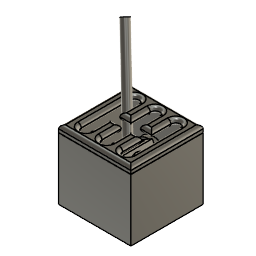
sim shifter v7 (Autodesk Fusion 360 design; units mm, degrees)
Autodesk Fusion 360 part; units mm, degrees
sketch "Sketch1" plane through (0, 0, 0) normal (1, 0, 0) x (0, 1, 0)
  line L0 (10, 18) -> (-10, 18)
  line L1 (-10, 18) -> (-10, 25)
  line L2 (10, 18) -> (10, 25)
  spline S0 degree 2 poles (-10, 25) (0, 18) (10, 25) knots 0 0 0 2.258871 2.258871 2.258871 weights 1 3 1
  line L3 (-22, 25) -> (-10, 25)
  line L4 (22, 25) -> (10, 25)
  line L5 (-16, 25) -> (-16, 20)
  line L6 (16, 25) -> (16, 20)
  spline S1 degree 2 poles (10, 25) (16, 20) (22, 25) knots 0 0 0 1.415097 1.415097 1.415097 weights 1 3 1
  spline S2 degree 2 poles (-22, 25) (-16, 20) (-10, 25) knots 0 0 0 1.415097 1.415097 1.415097 weights 1 3 1
  line L7 (-22, 11) -> (-25, 11)
  line L8 (-25, 11) -> (-25, 25)
  line L9 (-25, 25) -> (-22, 25)
  line L10 (22, 11) -> (22, 25)
  line L11 (-25, 25) -> (-20, 25)
  line L12 (0, 50) -> (0, 54)
  circle A0 centre (0, 50) radius 11
  circle A1 centre (0, 50) radius 4
  circle A2 centre (0, 14.836) radius 4
  line L13 (-22, 11) -> (-22, 25)
  line L14 (22, 11) -> (0, 11)
  line L15 (0, 11) -> (-22, 11)
  line L16 (22, 11) -> (25, 11)
  line L17 (25, 11) -> (25, 25)
  line L18 (25, 25) -> (22, 25)
  line L19 (22, 25) -> (22, 11)
  line L20 (0, 50) -> (7, 50)
  line L21 (7, 50) -> (7, 9.4684)
  line L22 (0, 50) -> (-7, 50)
  line L23 (-7, 50) -> (-7, 9.4684)
  line L24 (-7, 9.4684) -> (7, 9.4684)
  line L25 (-7, 50) -> (7, 50)
  line L26 (7, 50) -> (7, 70)
  line L27 (7, 70) -> (-7, 70)
  line L28 (-7, 70) -> (-7, 50)
  line L29 (-3.9999, 14.8053) -> (4.0001, 14.8053)
  line L30 (4.0001, 14.8053) -> (4.0001, 34.8053)
  line L31 (4.0001, 34.8053) -> (-3.9999, 34.8053)
  line L32 (-3.9999, 34.8053) -> (-3.9999, 14.8053)
  circle A3 centre (0.0001, 34.8053) radius 4
  line L33 (-25, 25) -> (-22, 25)
  line L34 (-22, 25) -> (-22, 65)
  line L35 (-22, 65) -> (-25, 65)
  line L36 (-25, 65) -> (-25, 25)
  line L37 (25, 25) -> (22, 25)
  line L38 (22, 25) -> (22, 65)
  line L39 (22, 65) -> (25, 65)
  line L40 (25, 65) -> (25, 25)
  line L41 (-22, 65) -> (22, 65)
  line L42 (22, 65) -> (22, 35.821)
  line L43 (22, 35.821) -> (-22, 35.821)
  line L44 (-22, 35.821) -> (-22, 65)
  dimension "d7" = 7
  dimension "d8" = 7
  dimension "d12" = 5
  dimension "d13" = 5
  dimension "d76" = 3
  dimension "d77" = 14
  dimension "d120" = 22
  dimension "d121" = 8
  dimension "d122" = 8
  dimension "d123" = 22
  dimension "d124" = 22
  dimension "d127" = 3
  dimension "d128" = 7
  dimension "d131" = 7
  dimension "d132" = 20
  dimension "d133" = 8
  dimension "d134" = 20
  dimension "d143" = 40
  dimension "d144" = 40
  constraint horizontal L0
  constraint perpendicular L0 L1
  constraint perpendicular L0 L2
  constraint perpendicular L1 L3
  constraint perpendicular L2 L4
  constraint midpoint L3 L5.start
  constraint perpendicular L3 L5
  constraint midpoint L4 L6.start
  constraint perpendicular L4 L6
  constraint perpendicular L3 L8
  constraint vertical L10
  constraint horizontal L11
  constraint coincident L12.start A0.centre
  constraint concentric A0 A1
  constraint perpendicular L9 L13
  constraint horizontal L14
  constraint perpendicular L10 L15
  constraint horizontal L16
  constraint vertical L17
  constraint horizontal L18
  constraint vertical L19
  constraint horizontal L20
  constraint vertical L21
  constraint perpendicular L12 L22
  constraint perpendicular L21 L24
  constraint horizontal L25
  constraint vertical L26
  constraint horizontal L27
  constraint vertical L28
  constraint horizontal L29
  constraint vertical L30
  constraint horizontal L31
  constraint vertical L32
  constraint coincident A2 L29.start
  constraint midpoint L31 A3.centre
  constraint coincident L30.end A3
  constraint horizontal L33
  constraint vertical L34
  constraint horizontal L35
  constraint vertical L36
  constraint horizontal L37
  constraint vertical L38
  constraint horizontal L39
  constraint vertical L40
  constraint horizontal L41
  constraint vertical L42
  constraint horizontal L43
  constraint vertical L44
  constraint coincident L38 L42.end
  measures "d7" distance of L0.end L1.end
  measures "d8" distance of L0.start L2.end
  measures "d12" distance of L5.start L5.end
  measures "d13" distance of L6.start L6.end
  measures "d76" distance of L7.start L7.end
  measures "d77" distance of L7.end L8.end
  measures "d120" diameter of A0
  measures "d121" diameter of A1
  measures "d122" diameter of A2
  measures "d123" distance of L10.start L14.end
  measures "d124" distance of L7.start L14.end
  measures "d127" distance of L10.start L16.end
  measures "d128" distance of L12.start L20.end
  measures "d131" distance of L12.start L22.end
  measures "d132" distance of L22.end L27.end
  measures "d133" distance of L29.start L29.end
  measures "d134" distance of L29.end L30.end
  measures "d143" distance of L8.end L35.end
  measures "d144" distance of L17.end L39.end
extrude "Extrude15" add sketch "Sketch1" along normal mid plane 20 contours A0 A1 L20 L21 L22 L23 L25 | A0 A1 L20 L22 L25 L26 L28 | A0 L26 L28 L41 | L26 L27 L28 L41 makes body 1
extrude "Extrude22" add sketch "Sketch1" along normal mid plane 10 contours L0 A2 L14 L21 L30 | L0 S0 L21 L30 | S0 L21 L30 A3 L43 | A2 L14 L15 L21 L23 L24 | L0 A2 L15 L23 L32 | A0 L21 L23 A3 L43 | L0 S0 L23 L32 | S0 L23 L32 A3 L43 bodies 1
extrude "Extrude16" add sketch "Sketch1" along normal mid plane 40 separate body contours L0 L2 S1 L10 L14 L19 L21 | L0 L2 S0 L21 | L0 A2 L14 L21 L30 | L0 S0 L21 L30 | L0 A2 L30 | L0 S0 A2 L30 L32 | L0 A2 L15 L23 L32 | L0 A2 L29 L30 | L0 A2 | L10 L16 L17 L18 L19 L37 | A2 L14 L15 L29 | L18 L37 L38 L39 L40 L42 | L0 A2 L32 | L0 S0 L23 L32 | L0 L1 S0 L23 | L0 L1 S2 L13 L15 L23 | L7 L8 L9 L11 L13 L33 | L9 L11 L33 L34 L35 L36 L44 makes body 2
extrude "Extrude17" cut sketch "Sketch1" along normal mid plane 20.4 contours L0 L2 S1 L10 L14 L19 L21 | L0 L2 S0 L21 | L0 A2 L14 L21 L30 | L0 S0 L21 L30 | L0 A2 L30 | L0 S0 A2 L30 L32 | L0 A2 L15 L23 L32 | L0 A2 L29 L30 | L0 A2 | A2 L14 L15 L29 | L0 A2 L32 | L0 S0 L23 L32 | L0 L1 S0 L23 | L0 L1 S2 L13 L15 L23 bodies 2
extrude "Extrude18" add sketch "Sketch1" along normal blind 10.2 and the other way blind -20 contours A0 L21 L23 A3 L43 | A0 L21 L26 L38 L41 L42 L43 | L18 L37 L38 L39 L40 L42 | A3 L43 | A0 L23 L28 L34 L41 L43 L44 | A0 L26 L28 L41 | L9 L11 L33 L34 L35 L36 L44 bodies 2
extrude "Extrude19" add sketch "Sketch1" along normal blind -10.2 and the other way blind 20 contours A0 L21 L23 A3 L43 | A0 L21 L26 L38 L41 L42 L43 | L18 L37 L38 L39 L40 L42 | A3 L43 | A0 L23 L28 L34 L41 L43 L44 | A0 L26 L28 L41 | L9 L11 L33 L34 L35 L36 L44 bodies 2
sketch "Sketch4" plane through (0, -25, 0) normal (0, -1, 0) x (1, 0, 0)
  circle A0 through (11, 50, -25) (-5.5, 59.5263, -25) (-5.5, 40.4737, -25)
  circle A1 through (20, 50, -25) (-10, 67.3205, -25) (-10, 32.6795, -25)
  circle A2 through (4, 50, -25) (-2, 53.4641, -25) (-2, 46.5359, -25)
  line L0 (0, 50, -25) -> (0, 25, -25)
  line L1 (0, 25, -25) -> (-20, 25, -25)
  line L2 (0, 25, -25) -> (20, 25, -25)
  line L3 (20, 25, -25) -> (45, 25, -25)
  line L4 (-20, 25, -25) -> (-45, 25, -25)
  line L5 (20, 25, -25) -> (30.6066, 35.6066, -25)
  line L6 (20, 25, -25) -> (35, 25, -25) construction
  line L7 (-20, 25, -25) -> (-30.6066, 35.6066, -25)
  line L8 (-20, 25, -25) -> (-35, 25, -25) construction
  spline S0 degree 5 poles (-45, 25, -25) (-44.3564, 25.3564, -25) (-43.0817, 26.0817, -25) (-41.2073, 27.2073, -25) (-38.7846, 28.7846, -25) (-35.8924, 30.8924, -25) (-33.1485, 33.1485, -25) (-30.565, 35.565, -25) (-28.1485, 38.1485, -25) (-25.8924, 40.8924, -25) (-23.7846, 43.7846, -25) (-22.2073, 46.2073, -25) (-21.0817, 48.0817, -25) (-20.3564, 49.3564, -25) (-20, 50, -25) knots 0 0 0 0 0 0 0.1 0.2 0.3 0.4 0.5 0.6 0.7 0.8 0.9 1 1 1 1 1 1
  spline S1 degree 5 poles (20, 50, -25) (20.3564, 49.3564, -25) (21.0817, 48.0817, -25) (22.2073, 46.2073, -25) (23.7846, 43.7846, -25) (25.8924, 40.8924, -25) (28.1485, 38.1485, -25) (30.565, 35.565, -25) (33.1485, 33.1485, -25) (35.8924, 30.8924, -25) (38.7846, 28.7846, -25) (41.2073, 27.2073, -25) (43.0817, 26.0817, -25) (44.3564, 25.3564, -25) (45, 25, -25) knots 0 0 0 0 0 0 0.1 0.2 0.3 0.4 0.5 0.6 0.7 0.8 0.9 1 1 1 1 1 1
  line L9 (45, 25, -25) -> (-45, 25, -25)
  line L10 (-45, 25, -25) -> (-45, 5, -25)
  line L11 (-45, 5, -25) -> (45, 5, -25)
  line L12 (45, 5, -25) -> (45, 25, -25)
  point P0 (0, 50)
  dimension "d153" = 22
  dimension "d154" = 8
  dimension "d155" = 25
  dimension "d156" = 90
  dimension "d157" = 25
  dimension "d159" = 15
  dimension "d160" = 45
  dimension "d161" = 45
  dimension "d162" = 15
  dimension "d171" = 90
  dimension "d172" = 20
extrude "Extrude20" add sketch "Sketch4" along normal blind 25.2 and the other way blind -32 separate body contours A1 | A1 L0 L2 L5 S1 L9 | A1 L0 L1 L7 S0 L9 | L3 L5 S1 L9 | L4 L7 S0 L9 | L1 L2 L3 L4 L9 L10 L11 L12 in plane through (0, 0, 0) normal (0, -1, 0) makes body 3
extrude "Extrude21" add sketch "Sketch4" along normal blind -25.2 and the other way blind 32 separate body contours A1 | A1 L0 L2 L5 S1 L9 | A1 L0 L1 L7 S0 L9 | L3 L5 S1 L9 | L4 L7 S0 L9 | L1 L2 L3 L4 L9 L10 L11 L12 in plane through (0, 0, 0) normal (0, -1, 0) makes body 4
extrude "Extrude23" add sketch "Sketch4" along normal blind 10 from surface at 32 contours L1 L2 L3 L4 L9 L10 L11 L12 in plane through (0, 0, 0) normal (0, -1, 0) bodies 3
extrude "Extrude24" add sketch "Sketch4" against normal blind 10 from surface at -32 contours L1 L2 L3 L4 L9 L10 L11 L12 in plane through (0, 0, 0) normal (0, -1, 0) bodies 4
sketch "Sketch5" plane through (0, 0, 25) normal (0, 0, 1) x (-1, 0, 0)
  line L0 (-45, 32, 10) -> (45, 32, 10)
  line L1 (45, 32, 10) -> (45, 42, 10)
  line L2 (45, 42, 10) -> (-45, 42, 10)
  line L3 (-45, 42, 10) -> (-45, 32, 10)
  line L4 (45, -32, 10) -> (-45, -32, 10)
  line L5 (-45, -32, 10) -> (-45, -42, 10)
  line L6 (-45, -42, 10) -> (45, -42, 10)
  line L7 (45, -42, 10) -> (45, -32, 10)
  line L8 (-45, 25.2, 10) -> (-20, 25.2, 10)
  line L9 (-20, 25.2, 10) -> (-20, 32, 10)
  line L10 (-45, 32, 10) -> (-20, 32, 10)
  line L11 (-45, 32, 10) -> (-45, 25.2, 10)
  line L12 (-20, -25.2, 10) -> (-45, -25.2, 10)
  line L13 (-45, -25.2, 10) -> (-45, -32, 10)
  line L14 (-20, -32, 10) -> (-45, -32, 10)
  line L15 (-20, -32, 10) -> (-20, -25.2, 10)
  line L16 (45, -25.2, 10) -> (20, -25.2, 10)
  line L17 (20, -25.2, 10) -> (20, -32, 10)
  line L18 (45, -32, 10) -> (20, -32, 10)
  line L19 (45, -32, 10) -> (45, -25.2, 10)
  line L20 (20, 25.2, 10) -> (45, 25.2, 10)
  line L21 (45, 25.2, 10) -> (45, 32, 10)
  line L22 (20, 32, 10) -> (45, 32, 10)
  line L23 (20, 32, 10) -> (20, 25.2, 10)
  line L24 (-45, -37, 10) -> (-35, -37, 10)
  line L25 (45, -37, 10) -> (35, -37, 10)
  line L26 (45, 37, 10) -> (35, 37, 10)
  line L27 (-45, 37, 10) -> (-35, 37, 10)
  line L28 (-45, 28.6, 10) -> (-35, 28.6, 10)
  line L29 (45, 28.6, 10) -> (35, 28.6, 10)
  line L30 (45, -28.6, 10) -> (35, -28.6, 10)
  line L31 (-45, -28.6, 10) -> (-35, -28.6, 10)
  dimension "d183" = 10
  dimension "d184" = 10
  dimension "d185" = 10
  dimension "d186" = 10
  dimension "d187" = 10
  dimension "d188" = 10
  dimension "d189" = 10
  dimension "d207" = 10
sketch "Sketch6" plane through (0, 0, 0) normal (0, 0, 1) x (1, 0, 0)
  line L0 (-45, -42) -> (45, -42)
  line L1 (45, -42) -> (45, -32)
  line L2 (45, -32) -> (-45, -32)
  line L3 (45, -32) -> (-45, -32)
  line L4 (-45, -32) -> (-45, -42)
  line L5 (-45, -42) -> (45, -42)
  line L6 (45, 42) -> (-45, 42)
  line L7 (-45, 42) -> (-45, 32)
  line L8 (-45, 32) -> (45, 32)
  line L9 (-45, 32) -> (45, 32)
  line L10 (45, 32) -> (45, 42)
  line L11 (45, 42) -> (-45, 42)
  line L12 (-45, 42) -> (45, 42)
  line L13 (45, 42) -> (45, -42)
  line L14 (45, -42) -> (-45, -42)
  line L15 (-45, -42) -> (-45, 42)
  line L16 (47.5, 47.5) -> (-47.5, 47.5)
  line L17 (-47.5, 47.5) -> (-47.5, -47.5)
  line L18 (-47.5, -47.5) -> (47.5, -47.5)
  line L19 (47.5, -47.5) -> (47.5, 47.5)
  line L20 (47.5, 47.5) -> (-47.5, -47.5) construction
  line L21 (-47.5, 47.5) -> (47.5, -47.5) construction
  line L22 (52.5, -52.5) -> (-52.5, -52.5)
  line L23 (-52.5, -52.5) -> (-52.5, 52.5)
  line L24 (-52.5, 52.5) -> (52.5, 52.5)
  line L25 (52.5, 52.5) -> (52.5, -52.5)
  line L26 (52.5, -52.5) -> (-52.5, 52.5) construction
  line L27 (-52.5, -52.5) -> (52.5, 52.5) construction
  line L28 (-45, -32) -> (-45, -42)
  line L29 (45, -42) -> (45, -32)
  line L30 (45, 32) -> (45, 42)
  line L31 (-45, 42) -> (-45, 32)
  dimension "d197" = 95
  dimension "d198" = 95
  dimension "d199" = 105
  dimension "d200" = 105
  constraint horizontal L12
  constraint vertical L13
  constraint horizontal L14
  constraint vertical L15
  constraint coincident L0.end L1.start
  constraint coincident L6.end L7.start
  constraint horizontal L16
  constraint perpendicular L16 L17
  constraint parallel L16 L18
  constraint parallel L17 L19
  constraint coincident L20 origin
  constraint coincident L21 origin
  constraint horizontal L22
  constraint perpendicular L22 L23
  constraint parallel L22 L24
  constraint parallel L23 L25
  constraint coincident L26 origin
  constraint coincident L27 origin
  measures "d197" distance of L17.end L18.end
  measures "d198" distance of L16.end L17.end
  measures "d199" distance of L23.end L24.end
  measures "d200" distance of L22.end L23.end
extrude "Extrude25" add sketch "Sketch6" along normal blind 5 separate body contours L0 L1 L2 L3 L4 L5 L13 L14 L15 L28 L29 | L2 L3 L8 L9 L13 L15 | L6 L7 L8 L9 L10 L11 L12 L13 L15 L30 L31 | L16 L17 L18 L19 | L22 L23 L24 L25 makes body 5
hole "Hole2" at (35, 37, 35) at (35, 28.6, 35) at (35, -28.6, 35) at (35, -37, 35) at (-35, -28.6, 35) at (-35, -37, 35) at (-35, 28.6, 35) at (-35, 37, 35) direction (0, 0, -1) diameter 2.529 depth 45 tip angle 118 counterbore diameter 10 counterbore depth 25 bodies 3 4 5
thread "Thread2" "ISO Metric profile 3.0 M3x0.5 M3x0.5 6H" major diameter 3.086 minor diameter 2.529 pitch 0.5 angle 60 resizes the face on face at (-35.7635, 27.592, 8.3333) on face at (34.2365, 27.592, 3.3333) on face at (-34.1872, 37.9687, 8.3333) on face at (34.2365, -29.608, 3.3333) on face at (35.8128, 37.9687, 3.3333) on face at (-35.7635, 27.592, 3.3333) on face at (-34.1872, -36.0313, 3.3333) on face at (-34.1872, 37.9687, 3.3333) on face at (35.8128, 37.9687, 8.3333) on face at (-35.7635, -29.608, 8.3333) on face at (34.2365, -29.608, 8.3333) on face at (34.2365, 27.592, 8.3333) on face at (-35.7635, -29.608, 3.3333) on face at (-34.1872, -36.0313, 8.3333) on face at (35.8128, -36.0313, 8.3333) on face at (35.8128, -36.0313, 3.3333) on bodies 3 4 5
fillet "Fillet1" radius 10 2 edges at (-20, 0, 11) (20, 0, 11) on bodies 2
extrude "Extrude26" add sketch "Sketch4" along normal mid plane 64 contours A2 in plane through (0, 0, 0) normal (0, -1, 0) bodies 2
extrude "Extrude27" cut sketch "Sketch4" along normal mid plane 44 contours A2 in plane through (0, 0, 0) normal (0, -1, 0) bodies 2
extrude "Extrude28" add sketch "Sketch6" along normal blind 90 contours L22 L23 L24 L25 bodies 5
sketch "Sketch7" plane through (0, 0, 0) normal (0, 0, 1) x (1, 0, 0)
  line L0 (52.5, 52.5) -> (-52.5, 52.5)
  line L1 (-52.5, 52.5) -> (-52.5, -52.5)
  line L2 (-52.5, -52.5) -> (52.5, -52.5)
  line L3 (52.5, -52.5) -> (52.5, 52.5)
  line L4 (0, 0) -> (0, 35)
  line L5 (0, 0) -> (0, -35)
  line L6 (0, 0) -> (30, 0)
  line L7 (30, 0) -> (30, 35)
  line L8 (0, 0) -> (-30, 0)
  line L9 (-30, 0) -> (-30, 35)
  line L10 (-30, 0) -> (-30, -35)
  line L11 (30, 0) -> (30, -35)
  circle A0 centre (-30, 35) radius 7
  circle A1 centre (-30, -35) radius 7
  circle A2 centre (0, -35) radius 7
  circle A3 centre (0, 35) radius 7
  circle A4 centre (30, 35) radius 7
  circle A5 centre (30, -35) radius 7
  line L12 (37, 35) -> (37, -35)
  line L13 (23, 35) -> (23, -35)
  line L14 (7, 35) -> (7, -35)
  line L15 (-7, 35) -> (-7, -35)
  line L16 (-23, -35) -> (-23, 35)
  line L17 (-37, 35) -> (-37, -35)
  circle A6 centre (-30, 0) radius 7
  circle A7 centre (30, 0) radius 7
  line L18 (30, 7) -> (-30, 7)
  line L19 (30, -7) -> (-30, -7)
  line L20 (30, -7) -> (37, -7)
  line L21 (30, 7) -> (37, 7)
  line L22 (-30, 7) -> (-37, 7)
  line L23 (-30, -7) -> (-37, -7)
  line L24 (-45, 45) -> (45, 45)
  line L25 (45, 45) -> (45, -45)
  line L26 (45, -45) -> (-45, -45)
  line L27 (-45, -45) -> (-45, 45)
  line L28 (-45, 45) -> (45, -45) construction
  line L29 (45, 45) -> (-45, -45) construction
  dimension "d210" = 35
  dimension "d211" = 35
  dimension "d212" = 30
  dimension "d213" = 30
  dimension "d214" = 35
  dimension "d215" = 35
  dimension "d216" = 35
  dimension "d217" = 14
  dimension "d218" = 14
  dimension "d219" = 14
  dimension "d220" = 14
  dimension "d221" = 14
  dimension "d222" = 14
  dimension "d223" = 35
  dimension "d228" = 90
  dimension "d229" = 90
  constraint coincident L4.start L5.start
  constraint parallel L4 L5
  constraint perpendicular L4 L6
  constraint perpendicular L6 L7
  constraint perpendicular L4 L8
  constraint perpendicular L8 L9
  constraint perpendicular L8 L10
  constraint perpendicular L6 L11
  constraint coincident L9.end A0.centre
  constraint coincident L10.end A1.centre
  constraint coincident L5.end A2.centre
  constraint coincident L4.end A3.centre
  constraint coincident L7.end A4.centre
  constraint coincident L11.end A5.centre
  constraint coincident A4 L12.start
  constraint coincident A5 L12.end
  constraint tangent A5 L12
  constraint parallel L7 L12
  constraint coincident A4 L13.start
  constraint coincident A5 L13.end
  constraint tangent A5 L13
  constraint perpendicular L6 L13
  constraint coincident A3 L14.start
  constraint coincident A2 L14.end
  constraint tangent A2 L14
  constraint parallel L4 L14
  constraint coincident A3 L15.start
  constraint coincident A2 L15.end
  constraint tangent A2 L15
  constraint parallel L4 L15
  constraint coincident A1 L16.start
  constraint coincident A0 L16.end
  constraint tangent A0 L16
  constraint perpendicular L8 L16
  constraint coincident A0 L17.start
  constraint coincident A1 L17.end
  constraint tangent A1 L17
  constraint parallel L9 L17
  constraint coincident L8.end L9.start
  constraint tangent L17 A6
  constraint coincident L6.end L7.start
  constraint tangent L13 A7
  constraint coincident A7 L18.start
  constraint coincident L7 L18.start
  constraint coincident A6 L18.end
  constraint coincident L9 L18.end
  constraint coincident A7 L19.start
  constraint coincident L11 L19.start
  constraint coincident L10 L19.end
  constraint coincident A6 L19.end
  constraint coincident L12 L20.end
  constraint tangent A7 L20
  constraint coincident L12 L21.end
  constraint tangent A7 L21
  constraint coincident L17 L22.end
  constraint tangent A6 L22
  constraint coincident L17 L23.end
  constraint tangent A6 L23
  constraint horizontal L24
  constraint perpendicular L24 L25
  constraint parallel L24 L26
  constraint parallel L25 L27
  constraint coincident L28 L4.start
  constraint coincident L29 L4.start
  measures "d210" distance of L4.start L4.end
  measures "d211" distance of L4.start L5.end
  measures "d212" distance of L4.start L6.end
  measures "d213" distance of L4.start L8.end
  measures "d214" distance of L8.end L9.end
  measures "d215" distance of L8.end L10.end
  measures "d216" distance of L6.end L11.end
  measures "d217" diameter of A0
  measures "d218" diameter of A1
  measures "d219" diameter of A2
  measures "d220" diameter of A3
  measures "d221" diameter of A4
  measures "d222" diameter of A5
  measures "d223" distance of L6.end L7.end
  measures "d228" distance of L25.end L26.end
  measures "d229" distance of L24.end L25.end
extrude "Extrude29" add sketch "Sketch7" along normal blind 90.2 and the other way blind -100 separate body contours L0 L1 L2 L3 | L24 L25 L26 L27 makes body 6
sketch "Sketch8" plane through (0, 0, 70) normal (0, 0, 1) x (-1, 0, 0)
  line L0 (-10, -7) -> (10, -7)
  line L1 (10, -7) -> (10, 7)
  line L2 (10, 7) -> (-10, 7)
  line L3 (-10, 7) -> (-10, -7)
  circle A0 centre (0, 0) radius 6
  dimension "d230" = 12
  constraint coincident A0.centre origin
  measures "d230" diameter of A0
extrude "Extrude30" add sketch "Sketch8" along normal blind 130 contours A0 bodies 1
move_body "Move2" bodies 2 1 to x (0.866025, 0, 0.5) y (0, 1, 0) z (-0.5, 0, 0.866025) at (21.1762, 0, 6.6758)
fillet "Fillet2" radius 5 1 faces at (-47.3333, 0, 100) on bodies 6
fillet "Fillet3" radius 5 20 edges at (15, -7, 90.2) (15, 7, 90.2) (-7, 21, 90.2) (0, 42, 90.2) (7, 21, 90.2) (7, -21, 90.2) (0, -42, 90.2) (-7, -21, 90.2) (23, 21, 90.2) (30, 42, 90.2) (37, 0, 90.2) (30, -42, 90.2) (23, -21, 90.2) (-15, 7, 90.2) (-15, -7, 90.2) (-23, -21, 90.2) (-30, -42, 90.2) (-37, 0, 90.2) (-30, 42, 90.2) (-23, 21, 90.2) on bodies 6
move_body "Move3" bodies 1 to x (0.976577, -0.211309, 0.04057) y (0.211309, 0.906308, -0.365998) z (0.04057, 0.365998, 0.929731) at (-2.1171, -19.0995, 3.667)
